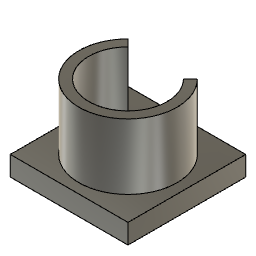
12mm hose holder (Autodesk Fusion 360 design; units mm, degrees)
Autodesk Fusion 360 part; units mm, degrees
sketch "Sketch12" plane through (0, 0, 0) normal (0, 0, 1) x (1, 0, 0)
  line L0 (9, 9) -> (-9, 9)
  line L1 (-9, 9) -> (-9, -9)
  line L2 (-9, -9) -> (9, -9)
  line L3 (9, -9) -> (9, 9)
  line L4 (9, 9) -> (-9, -9) construction
  line L5 (-9, 9) -> (9, -9) construction
  dimension "d31" = 18
  dimension "d32" = 18
  constraint horizontal L0
  constraint perpendicular L0 L1
  constraint parallel L0 L2
  constraint parallel L1 L3
  constraint coincident L4 origin
  constraint coincident L5 origin
  measures "d31" distance of L0.start L0.end
  measures "d32" distance of L0.end L1.end
extrude "Extrude6" add sketch "Sketch12" along normal blind 3
sketch "Sketch13" plane through (0, 0, 3) normal (0, 0, 1) x (-1, 0, 0)
  line L0 (-9, 9) -> (-9, -9)
  line L1 (-9, -9) -> (9, -9)
  line L2 (9, -9) -> (9, 9)
  line L3 (9, 9) -> (-9, 9)
  line L4 (4.2426, -4.2426) -> (5.3033, -5.3033)
  line L5 (-4.2426, -4.2426) -> (-5.3033, -5.3033)
  line L6 (15, 0) -> (-21.4677, 0) construction
  arc A0 (5.3033, -5.3033) -> (-5.3033, -5.3033) centre (0, 0) ccw
  arc A1 (4.2426, -4.2426) -> (-4.2426, -4.2426) centre (0, 0) ccw
  dimension "d35" = 15
  dimension "d36" = 12
  dimension "d37" = 90
  dimension "d38" = 45
  constraint coincident A0.centre A1.centre
  constraint perpendicular L4 L5
  constraint horizontal L6
  measures "d35" diameter of A0
  measures "d36" diameter of A1
  measures "d37" angle of L4 L5
  measures "d38" angle of L4 L6
extrude "Extrude7" add sketch "Sketch13" along normal blind 10 contours L4 L5 A0 A1
sketch "Sketch7" plane through (0, 0, 0) normal (0, 1, 0) x (1, 0, 0)
sketch "Sketch6" plane through (0, 0, 0) normal (0, 0, 1) x (1, 0, 0)
  line L0 (0, 18) -> (18, 18)
  line L1 (18, 18) -> (18, 0)
  line L2 (18, 0) -> (0, 0)
  line L3 (0, 0) -> (0, 18)
  line L4 (4.4239, 12.7997) -> (3.65, 13.433)
  line L5 (13.711, 12.7997) -> (14.4849, 13.433)
  arc A0 (4.4239, 12.7997) -> (13.711, 12.7997) centre (9.0674, 9) ccw
  arc A1 (3.65, 13.433) -> (14.4849, 13.433) centre (9.0674, 9) ccw
  dimension "d11" = 18
  dimension "d12" = 18
  dimension "d13" = 14
  dimension "d14" = 12
  constraint horizontal L0
  constraint vertical L1
  constraint horizontal L2
  constraint vertical L3
  constraint coincident L2.end L3.start
  constraint concentric A0 A1
  measures "d11" distance of L0.start L0.end
  measures "d12" distance of L0.end L1.end
  measures "d13" diameter of A1
  measures "d14" diameter of A0
sketch "Sketch1" plane through (0, 0, 0) normal (0, 1, 0) x (1, 0, 0)
  line L0 (0, -25) -> (20, -25)
  line L1 (20, -25) -> (20, -5)
  line L2 (20, -5) -> (0, -5)
  line L3 (0, -5) -> (0, -25)
  dimension "d1" = 20
  dimension "d2" = 20
  constraint horizontal L0
  constraint vertical L1
  constraint horizontal L2
  constraint vertical L3
  measures "d1" distance of L0.start L2.end
  measures "d2" distance of L0.start L0.end
sketch "Sketch2" plane through (0, 0, 0) normal (0, 1, 0) x (1, 0, 0)
extrude "Extrude1" [rolled back] along distance 4 taper angle 0
extrude "Extrude2" [rolled back] along distance -2.5 taper angle 0
sketch "Sketch3" plane through (0, 0, 0) normal (0, 1, 0) x (1, 0, 0)
  circle A0 centre (10, -15) radius 6
  circle A1 centre (10, -15) radius 7.5
  dimension "d7" = 12
  dimension "d8" = 15
  constraint concentric A0 A1
  measures "d7" diameter of A0
  measures "d8" diameter of A1
extrude "Extrude3" [rolled back] along distance -5 taper angle 0
sketch "Sketch4" plane through (0, -5, 0) normal (0, -1, 0) x (1, 0, 0)
combine "Combine1" [rolled back]
combine "Combine2" [rolled back]
